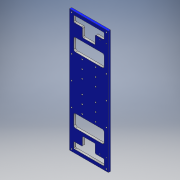
# Autodesk Inventor part: base_roulante
Saved by Autodesk Inventor 2017 (Build 210142000, 142)
## iProperties
Created: 2017-04-12
Part Number: base_roulante
Material: Generic
Document SubType Name: Modeling
Designer: franc
Density: 1 g/cm^3
Appearance: Default
Author: franc
Autodesk Inventor part; units mm, degrees
ref_plane "YZ Plane" through (0, 0, 0) normal (1, 0, 0) x (0, 1, 0)
ref_plane "XZ Plane" through (0, 0, 0) normal (0, 1, 0) x (-1, 0, 0)
ref_plane "XY Plane" through (0, 0, 0) normal (0, 0, 1) x (1, 0, 0)
sketch "Sketch1" plane through (0, 0, 0) normal (0, 1, 0) x (-1, 0, 0)
  line L0 (4.6641, 6.6919) -> (-87.3359, 6.6919)
  line L1 (-87.3359, 6.6919) -> (-87.3359, -283.3081)
  line L2 (-87.3359, -283.3081) -> (4.6641, -283.3081)
  line L3 (4.6641, -283.3081) -> (4.6641, 6.6919)
  point P0 (0, 0)
  dimension "d0" = 290
  dimension "d1" = 92
  constraints: 8 end point, 2 parallel, 1 horizontal, 1 perpendicular
  measures "d0" distance of L2.end L0.start
  measures "d1" distance of L0.start L0.end
extrude "Extrusion1" add sketch "Sketch1" along normal blind 5
sketch "Sketch2" plane through (0, 5, 0) normal (0, 1, 0) x (1, 0, 0)
  line L0 (-4.6641, 283.3081) -> (-4.6641, -6.6919) projected
  line L1 (87.3359, -6.6919) -> (87.3359, 283.3081) projected
  line L2 (9.3359, 45.3081) -> (73.3359, 45.3081)
  line L3 (77.3359, 49.3081) -> (77.3359, 71.3081)
  line L4 (73.3359, 75.3081) -> (9.3359, 75.3081)
  line L5 (5.3359, 71.3081) -> (5.3359, 49.3081)
  line L6 (-4.6641, -6.6919) -> (87.3359, -6.6919) projected
  arc A0 (5.3359, 49.3081) -> (9.3359, 45.3081) centre (9.3359, 49.3081) ccw
  arc A1 (9.3359, 75.3081) -> (5.3359, 71.3081) centre (9.3359, 71.3081) ccw
  arc A2 (77.3359, 71.3081) -> (73.3359, 75.3081) centre (73.3359, 71.3081) ccw
  arc A3 (73.3359, 45.3081) -> (77.3359, 49.3081) centre (73.3359, 49.3081) ccw
  line L7 (9.3359, 201.3081) -> (73.3359, 201.3081)
  line L8 (77.3359, 205.3081) -> (77.3359, 227.3081)
  line L9 (73.3359, 231.3081) -> (9.3359, 231.3081)
  line L10 (5.3359, 227.3081) -> (5.3359, 205.3081)
  arc A4 (5.3359, 205.3081) -> (9.3359, 201.3081) centre (9.3359, 205.3081) ccw
  arc A5 (9.3359, 231.3081) -> (5.3359, 227.3081) centre (9.3359, 227.3081) ccw
  arc A6 (77.3359, 227.3081) -> (73.3359, 231.3081) centre (73.3359, 227.3081) ccw
  arc A7 (73.3359, 201.3081) -> (77.3359, 205.3081) centre (73.3359, 205.3081) ccw
  line L11 (7.3359, 1.3081) -> (75.3359, 1.3081)
  line L12 (77.3359, 3.3081) -> (77.3359, 14.3081)
  line L13 (75.3359, 16.3081) -> (58.3359, 16.3081)
  line L14 (56.3359, 18.3081) -> (56.3359, 35.3081)
  line L15 (54.3359, 37.3081) -> (28.3359, 37.3081)
  line L16 (26.3359, 35.3081) -> (26.3359, 18.3081)
  line L17 (24.3359, 16.3081) -> (7.3359, 16.3081)
  line L18 (5.3359, 14.3081) -> (5.3359, 3.3081)
  arc A8 (5.3359, 3.3081) -> (7.3359, 1.3081) centre (7.3359, 3.3081) ccw
  arc A9 (7.3359, 16.3081) -> (5.3359, 14.3081) centre (7.3359, 14.3081) ccw
  arc A10 (24.3359, 16.3081) -> (26.3359, 18.3081) centre (24.3359, 18.3081) ccw
  arc A11 (28.3359, 37.3081) -> (26.3359, 35.3081) centre (28.3359, 35.3081) ccw
  arc A12 (56.3359, 35.3081) -> (54.3359, 37.3081) centre (54.3359, 35.3081) ccw
  arc A13 (56.3359, 18.3081) -> (58.3359, 16.3081) centre (58.3359, 18.3081) ccw
  arc A14 (77.3359, 14.3081) -> (75.3359, 16.3081) centre (75.3359, 14.3081) ccw
  arc A15 (75.3359, 1.3081) -> (77.3359, 3.3081) centre (75.3359, 3.3081) ccw
  line L19 (87.3359, 283.3081) -> (-4.6641, 283.3081) projected
  line L20 (5.3359, 273.3081) -> (5.3359, 262.3081)
  line L21 (7.3359, 260.3081) -> (24.3359, 260.3081)
  line L22 (26.3359, 258.3081) -> (26.3359, 241.3081)
  line L23 (28.3359, 239.3081) -> (54.3359, 239.3081)
  line L24 (56.3359, 241.3081) -> (56.3359, 258.3081)
  line L25 (58.3359, 260.3081) -> (75.3359, 260.3081)
  line L26 (77.3359, 262.3081) -> (77.3359, 273.3081)
  line L27 (75.3359, 275.3081) -> (7.3359, 275.3081)
  arc A16 (26.3359, 258.3081) -> (24.3359, 260.3081) centre (24.3359, 258.3081) ccw
  arc A17 (5.3359, 262.3081) -> (7.3359, 260.3081) centre (7.3359, 262.3081) ccw
  arc A18 (7.3359, 275.3081) -> (5.3359, 273.3081) centre (7.3359, 273.3081) ccw
  arc A19 (77.3359, 273.3081) -> (75.3359, 275.3081) centre (75.3359, 273.3081) ccw
  arc A20 (75.3359, 260.3081) -> (77.3359, 262.3081) centre (75.3359, 262.3081) ccw
  arc A21 (58.3359, 260.3081) -> (56.3359, 258.3081) centre (58.3359, 258.3081) ccw
  arc A22 (54.3359, 239.3081) -> (56.3359, 241.3081) centre (54.3359, 241.3081) ccw
  arc A23 (26.3359, 241.3081) -> (28.3359, 239.3081) centre (28.3359, 241.3081) ccw
  point P0 (5.3359, 45.3081)
  point P1 (77.3359, 75.3081)
  point P2 (5.3359, 75.3081)
  point P3 (5.3359, 201.3081)
  point P4 (77.3359, 201.3081)
  point P5 (5.3359, 231.3081)
  point P6 (5.3359, 1.3081)
  point P7 (77.3359, 1.3081)
  point P8 (77.3359, 16.3081)
  point P9 (56.3359, 16.3081)
  point P10 (26.3359, 16.3081)
  point P11 (5.3359, 16.3081)
  point P12 (5.3359, 275.3081)
  point P13 (5.3359, 260.3081)
  point P14 (26.3359, 260.3081)
  point P15 (56.3359, 260.3081)
  point P16 (77.3359, 260.3081)
  point P17 (77.3359, 275.3081)
  dimension "d12" = 30
  dimension "d13" = 72
  dimension "d14" = 10
  dimension "d16" = 4
  dimension "d17" = 30
  dimension "d18" = 10
  dimension "d19" = 72
  dimension "d21" = 4
  dimension "d41" = 10
  dimension "d42" = 72
  dimension "d43" = 15
  dimension "d44" = 21
  dimension "d45" = 21
  dimension "d46" = 36
  dimension "d47" = 15
  dimension "d48" = 8
  dimension "d49" = 2
  dimension "d58" = 10
  dimension "d59" = 8
  dimension "d60" = 72
  dimension "d61" = 15
  dimension "d62" = 36
  dimension "d63" = 21
  dimension "d64" = 21
  dimension "d65" = 2
  dimension "d66" = 2
  dimension "d170" = 8
  dimension "d171" = 8
  constraints: 48 end point, 48 point on circle, 48 tangent, 38 point on line, 24 centre point, 19 equal radius, 15 perpendicular, 4 parallel, 3 horizontal, 1 vertical
  measures "d12" distance of point (5.336, 75.308) point (5.336, 45.308)
  measures "d13" distance of point (77.336, 75.308) point (5.336, 75.308)
  measures "d14" distance between parallel lines of L0 L5
  measures "d16" radius of A0
  measures "d17" distance of point (5.336, 231.308) point (5.336, 201.308)
  measures "d18" distance between parallel lines of L0 L10
  measures "d19" distance of point (5.336, 201.308) point (77.336, 201.308)
  measures "d21" radius of A4
  measures "d41" distance between parallel lines of L0 L18
  measures "d42" distance of point (5.336, 1.308) point (77.336, 1.308)
  measures "d43" distance of point (77.336, 1.308) point (77.336, 16.308)
  measures "d44" distance of point (77.336, 16.308) point (56.336, 16.308)
  measures "d45" distance of point (26.336, 16.308) point (5.336, 16.308)
  measures "d46" distance between parallel lines of L15 L11
  measures "d47" distance of point (5.336, 16.308) point (5.336, 1.308)
  measures "d48" distance between parallel lines of L6 L11
  measures "d49" radius of A8
  measures "d58" distance between parallel lines of L0 L20
  measures "d59" distance between parallel lines of L19 L27
  measures "d60" distance of point (77.336, 275.308) point (5.336, 275.308)
  measures "d61" distance of point (77.336, 260.308) point (77.336, 275.308)
  measures "d62" distance between parallel lines of L27 L23
  measures "d63" distance of point (56.336, 260.308) point (77.336, 260.308)
  measures "d64" distance of point (5.336, 260.308) point (26.336, 260.308)
  measures "d65" radius of A16
  measures "d66" radius of A20
  measures "d170" distance between parallel lines of L23 L9
  measures "d171" distance between parallel lines of L15 L2
extrude "Extrusion2" cut sketch "Sketch2" against normal up to next contours A0 L5 A1 L4 A2 L3 A3 L2 | A4 L10 A5 L9 A6 L8 A7 L7 | A8 L18 A9 L17 A10 L16 A11 L15 A12 L14 A13 L13 A14 L12 A15 L11 | A18 L27 A19 L26 A20 L25 A21 L24 A22 L23 A23 L22 A16 L21 A17 L20
sketch "Sketch3" plane through (0, 5, 0) normal (0, 1, 0) x (1, 0, 0)
  circle A0 centre (0.3359, -1.6919) radius 1.5
  circle A1 centre (82.3359, -1.6919) radius 1.5
  circle A2 centre (0.3359, 83.3081) radius 1.5
  circle A3 centre (0.3359, 138.3081) radius 1.5
  circle A4 centre (0.3359, 193.3081) radius 1.5
  circle A5 centre (0.3359, 278.3081) radius 1.5
  circle A6 centre (82.3359, 83.3081) radius 1.5
  circle A7 centre (82.3359, 138.3081) radius 1.5
  circle A8 centre (82.3359, 193.3081) radius 1.5
  circle A9 centre (82.3359, 278.3081) radius 1.5
  line L0 (-4.6641, -6.6919) -> (87.3359, -6.6919) projected
  line L1 (-4.6641, 283.3081) -> (-4.6641, -6.6919) projected
  line L2 (87.3359, -6.6919) -> (87.3359, 283.3081) projected
  line L3 (87.3359, 283.3081) -> (-4.6641, 283.3081) projected
  circle A10 centre (82.3359, 21.3081) radius 1
  circle A11 centre (67.3359, 21.3081) radius 1
  circle A12 centre (82.3359, 255.3081) radius 1
  circle A13 centre (67.3359, 255.3081) radius 1
  circle A14 centre (25.3359, 82.3081) radius 1.5
  circle A15 centre (25.3359, 102.3081) radius 1.5
  circle A16 centre (57.3359, 82.3081) radius 1.5
  circle A17 centre (57.3359, 102.3081) radius 1.5
  circle A18 centre (25.3359, 194.3081) radius 1.5
  circle A19 centre (25.3359, 174.3081) radius 1.5
  circle A20 centre (57.3359, 194.3081) radius 1.5
  circle A21 centre (57.3359, 174.3081) radius 1.5
  line L4 (9.3359, 75.3081) -> (73.3359, 75.3081) projected
  line L5 (73.3359, 201.3081) -> (9.3359, 201.3081) projected
  circle A22 centre (57.3359, 122.3081) radius 1.5
  circle A23 centre (25.3359, 122.3081) radius 1.5
  circle A24 centre (25.3359, 154.3081) radius 1.5
  circle A25 centre (57.3359, 154.3081) radius 1.5
  line L6 (75.3359, 260.3081) -> (58.3359, 260.3081) projected
  line L7 (58.3359, 16.3081) -> (75.3359, 16.3081) projected
  point P0 (0, 0)
  dimension "d70" = 3
  dimension "d71" = 5
  dimension "d72" = 5
  dimension "d73" = 3
  dimension "d74" = 5
  dimension "d75" = 5
  dimension "d77" = 3
  dimension "d78" = 3
  dimension "d79" = 3
  dimension "d81" = 3
  dimension "d82" = 3
  dimension "d84" = 3
  dimension "d85" = 3
  dimension "d86" = 3
  dimension "d89" = 5
  dimension "d90" = 5
  dimension "d91" = 5
  dimension "d93" = 5
  dimension "d95" = 5
  dimension "d96" = 5
  dimension "d97" = 5
  dimension "d99" = 5
  dimension "d100" = 5
  dimension "d101" = 5
  dimension "d106" = 145
  dimension "d107" = 145
  dimension "d108" = 90
  dimension "d109" = 90
  dimension "d110" = 90
  dimension "d111" = 90
  dimension "d112" = 2
  dimension "d113" = 2
  dimension "d114" = 2
  dimension "d115" = 2
  dimension "d116" = 5
  dimension "d119" = 20
  dimension "d120" = 5
  dimension "d121" = 20
  dimension "d124" = 3
  dimension "d125" = 3
  dimension "d127" = 3
  dimension "d128" = 3
  dimension "d131" = 3
  dimension "d132" = 3
  dimension "d133" = 3
  dimension "d134" = 3
  dimension "d136" = 30
  dimension "d137" = 30
  dimension "d139" = 30
  dimension "d140" = 30
  dimension "d143" = 30
  dimension "d144" = 30
  dimension "d145" = 30
  dimension "d146" = 30
  dimension "d148" = 7
  dimension "d149" = 7
  dimension "d150" = 7
  dimension "d151" = 7
  dimension "d152" = 20
  dimension "d153" = 3
  dimension "d154" = 30
  dimension "d155" = 20
  dimension "d156" = 20
  dimension "d157" = 3
  constraints: 26 centre point
  measures "d70" diameter of A0
  measures "d71" distance from line of L0 A0.centre
  measures "d72" distance from line of L1 A0.centre
  measures "d73" diameter of A1
  measures "d74" distance from line of L0 A1.centre
  measures "d75" distance from line of L2 A1.centre
  measures "d77" diameter of A2
  measures "d78" diameter of A3
  measures "d79" diameter of A4
  measures "d81" diameter of A5
  measures "d82" diameter of A9
  measures "d84" diameter of A8
  measures "d85" diameter of A7
  measures "d86" diameter of A6
  measures "d89" distance from line of L1 A2.centre
  measures "d90" distance from line of L1 A3.centre
  measures "d91" distance from line of L1 A4.centre
  measures "d93" distance from line of L1 A5.centre
  measures "d95" distance from line of L2 A6.centre
  measures "d96" distance from line of L2 A7.centre
  measures "d97" distance from line of L2 A8.centre
  measures "d99" distance from line of L2 A9.centre
  measures "d100" distance from line of L3 A9.centre
  measures "d101" distance from line of L3 A5.centre
  measures "d106" distance from line of L0 A3.centre
  measures "d107" distance from line of L0 A7.centre
  measures "d108" distance from line of L3 A8.centre
  measures "d109" distance from line of L0 A6.centre
  measures "d110" distance from line of L3 A4.centre
  measures "d111" distance from line of L0 A2.centre
  measures "d112" diameter of A11
  measures "d113" diameter of A10
  measures "d114" diameter of A13
  measures "d115" diameter of A12
  measures "d116" distance from line of L2 A10.centre
  measures "d119" distance from line of L2 A11.centre
  measures "d120" distance from line of L2 A12.centre
  measures "d121" distance from line of L2 A13.centre
  measures "d124" diameter of A14
  measures "d125" diameter of A15
  measures "d127" diameter of A16
  measures "d128" diameter of A17
  measures "d131" diameter of A19
  measures "d132" diameter of A18
  measures "d133" diameter of A20
  measures "d134" diameter of A21
  measures "d136" distance from line of L2 A16.centre
  measures "d137" distance from line of L2 A17.centre
  measures "d139" distance from line of L1 A14.centre
  measures "d140" distance from line of L1 A15.centre
  measures "d143" distance from line of L1 A19.centre
  measures "d144" distance from line of L1 A18.centre
  measures "d145" distance from line of L2 A20.centre
  measures "d146" distance from line of L2 A21.centre
  measures "d148" distance from line of L4 A16.centre
  measures "d149" distance from line of L4 A14.centre
  measures "d150" distance from line of L5 A18.centre
  measures "d151" distance from line of L5 A20.centre
  measures "d152" distance of A17.centre A16.centre
  measures "d153" diameter of A22
  measures "d154" distance from line of L2 A22.centre
  measures "d155" distance of A22.centre A17.centre
  measures "d156" distance of A15.centre A14.centre
  measures "d157" diameter of A23
extrude "Extrusion3" cut sketch "Sketch3" against normal blind 5 contours A0 | A1 | A2 | A3 | A4 | A5 | A6 | A7 | A8 | A9 | A10 | A11 | A12 | A13 | A14 | A15 | A16 | A17 | A18 | A19 | A20 | A21 | A22 | A23 | A24 | A25
body "Solid1"
